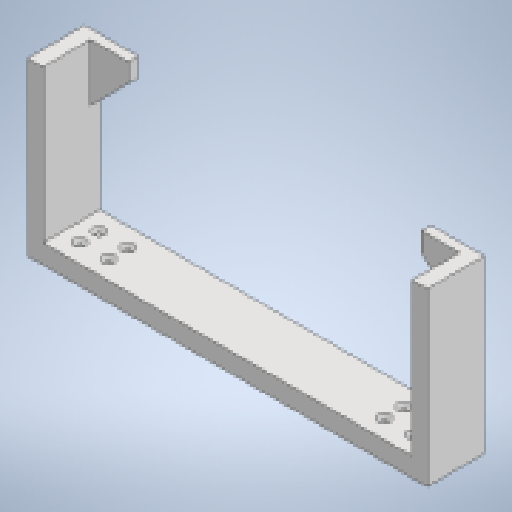
# Autodesk Inventor part: gantry_L
Saved by Autodesk Inventor 2024 (Build 280153000, 153)
## iProperties
Created: 2023-08-11
Part Number: gantry_L
Material: Generic
Document SubType Name: Modeling
Designer: l1534
Density: 1 g/cm^3
Appearance: Default
Author: l1534
Autodesk Inventor part; units mm, degrees
ref_plane "YZ Plane" through (0, 0, 0) normal (1, 0, 0) x (0, 1, 0)
ref_plane "XZ Plane" through (0, 0, 0) normal (0, 1, 0) x (-1, 0, 0)
ref_plane "XY Plane" through (0, 0, 0) normal (0, 0, 1) x (1, 0, 0)
sketch "Sketch1" plane through (0, 0, 0) normal (0, 0, 1) x (1, 0, 0)
  line L0 (-75.4115, 94.0727) -> (134.5885, 94.0727)
  line L1 (134.5885, 94.0727) -> (134.5885, 4.0727)
  line L2 (134.5885, 4.0727) -> (-75.4115, 4.0727)
  line L3 (-75.4115, 4.0727) -> (-75.4115, 94.0727)
  point P0 (0, 0)
  dimension "d0" = 210
  dimension "d1" = 90
  constraints: 8 end point, 2 parallel, 1 horizontal, 1 perpendicular
  measures "d0" distance of L0.start L0.end
  measures "d1" distance of L0.end L1.end
extrude "Extrusion1" add sketch "Sketch1" along normal blind 30
sketch "Sketch2" plane through (0, 0, 30) normal (0, 0, 1) x (1, 0, 0)
  line L0 (134.5885, 94.0727) -> (-75.4115, 94.0727) projected
  line L1 (-67.4115, 94.0727) -> (126.5885, 94.0727)
  line L2 (126.5885, 94.0727) -> (126.5885, 14.0727)
  line L3 (126.5885, 14.0727) -> (-67.4115, 14.0727)
  line L4 (-67.4115, 14.0727) -> (-67.4115, 94.0727)
  line L5 (-75.4115, 94.0727) -> (-75.4115, 4.0727) projected
  line L6 (134.5885, 4.0727) -> (134.5885, 94.0727) projected
  line L7 (-75.4115, 4.0727) -> (134.5885, 4.0727) projected
  point P0 (0, 0)
  dimension "d4" = 8
  dimension "d5" = 8
  dimension "d6" = 10
  constraints: 8 end point, 2 parallel, 1 horizontal, 1 perpendicular, 1 point on line
  measures "d4" distance between parallel lines of L5 L4
  measures "d5" distance between parallel lines of L6 L2
  measures "d6" distance between parallel lines of L7 L3
extrude "Extrusion2" cut sketch "Sketch2" against normal blind 30 contours L2 L3 L4 L0
sketch "Sketch3" plane through (-67.4115, 14.0727, 30) normal (0, 1, 0) x (1, 0, 0)
  circle A0 centre (9.5, 10) radius 1.5
  circle A1 centre (9.5, 20) radius 1.5
  circle A2 centre (24.5, 10) radius 1.5
  circle A3 centre (24.5, 20) radius 1.5
  circle A4 centre (184.5, 20) radius 1.5
  circle A5 centre (169.5, 10) radius 1.5
  circle A6 centre (184.5, 10) radius 1.5
  circle A7 centre (169.5, 20) radius 1.5
  line L0 (194, 0) -> (0, 0) projected
  line L1 (194, 30) -> (194, 0) projected
  point P0 (67.4115, 30)
  dimension "d9" = 3
  dimension "d10" = 3
  dimension "d11" = 3
  dimension "d12" = 3
  dimension "d13" = 3
  dimension "d14" = 3
  dimension "d15" = 3
  dimension "d16" = 3
  dimension "d18" = 10
  dimension "d19" = 10
  dimension "d20" = 10
  dimension "d21" = 10
  dimension "d22" = 15
  dimension "d23" = 15
  dimension "d24" = 9.5
  dimension "d25" = 15
  dimension "d26" = 15
  dimension "d27" = 9.5
  dimension "d28" = 10
  dimension "d29" = 10
  dimension "d30" = 10
  dimension "d31" = 10
  dimension "d33" = 145
  dimension "d34" = 145
  constraints: 8 centre point
  measures "d9" diameter of A0
  measures "d10" diameter of A1
  measures "d11" diameter of A2
  measures "d12" diameter of A3
  measures "d13" diameter of A6
  measures "d14" diameter of A7
  measures "d15" diameter of A5
  measures "d16" diameter of A4
  measures "d18" distance from line of L0 A6.centre
  measures "d19" distance from line of L0 A2.centre
  measures "d20" distance from line of L0 A0.centre
  measures "d21" distance from line of L0 A5.centre
  measures "d22" distance of A2.centre A0.centre
  measures "d23" distance of A3.centre A1.centre
  measures "d24" distance from line of L1 A6.centre
  measures "d25" distance of A6.centre A5.centre
  measures "d26" distance of A7.centre A4.centre
  measures "d27" distance from line of L1 A4.centre
  measures "d28" distance of A4.centre A6.centre
  measures "d29" distance of A5.centre A7.centre
  measures "d30" distance of A2.centre A3.centre
  measures "d31" distance of A0.centre A1.centre
  measures "d33" distance of A5.centre A2.centre
  measures "d34" distance of A7.centre A3.centre
extrude "Extrusion3" cut sketch "Sketch3" against normal blind 30
chamfer "Chamfer1" distance 1.8 angle 45 8 edges at (-59.4115, 14.0727, 10) (-59.4115, 14.0727, 20) (-44.4115, 14.0727, 20) (-44.4115, 14.0727, 10) (115.5885, 14.0727, 10) (115.5885, 14.0727, 20) (100.5885, 14.0727, 20) (100.5885, 14.0727, 10)
sketch "Sketch6" plane through (134.5885, 94.0727, 30) normal (0, 1, 0) x (1, 0, 0)
  line L0 (-8, 30) -> (-8, 0) projected
  line L1 (-8, 30) -> (-28, 30)
  line L2 (-28, 30) -> (-28, 25)
  line L3 (-28, 25) -> (-8, 25)
  line L4 (-8, 25) -> (-8, 30)
  line L5 (-210, 30) -> (0, 30) projected
  line L6 (-202, 30) -> (-182, 30)
  line L7 (-182, 30) -> (-182, 25)
  line L8 (-182, 25) -> (-202, 25)
  line L9 (-202, 25) -> (-202, 30)
  line L10 (-210, 30) -> (-210, 0) projected
  point P0 (-134.5885, 30)
  point P1 (-8, 25)
  dimension "d49" = 5
  dimension "d50" = 20
  dimension "d51" = 8
  dimension "d52" = 20
  constraints: 16 end point, 4 parallel, 2 horizontal, 2 perpendicular, 2 point on line
  measures "d49" distance of L6.end L7.end
  measures "d50" distance of L7.end L8.end
  measures "d51" distance between parallel lines of L10 L9
  measures "d52" distance of L2.end L3.end
extrude "Extrusion6" add sketch "Sketch6" against normal blind 10
chamfer "Chamfer2" distance 20 angle 45 2 edges at (126.5885, 84.0727, 2.5) (-67.4115, 84.0727, 2.5)
equation "\"d20\" = d19"
equation "\"d21\" = d18"
equation "\"d23\" = d22"
equation "\"d26\" = d25"
equation "\"d27\" = d24"
equation "\"d29\" = d28"
equation "\"d30\" = d29"
equation "\"d31\" = d30"
equation "\"d34\" = d33"
body "Solid1"
